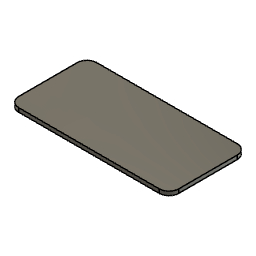
VFD_NTP_CLOCK_PLATE_T_V1.0 v3 (Autodesk Fusion 360 design; units mm, degrees)
Autodesk Fusion 360 part; units mm, degrees
sketch "スケッチ1" plane through (0, 0, 0) normal (0, 1, 0) x (1, 0, 0)
  line L0 (-41, 15) -> (-41, -15)
  line L1 (-36, 20) -> (36, 20)
  line L2 (41, 15) -> (41, -15)
  line L3 (-36, -20) -> (36, -20)
  arc A0 (-41, -15) -> (-36, -20) centre (-36, -15) ccw
  arc A1 (-36, 20) -> (-41, 15) centre (-36, 15) ccw
  arc A2 (41, 15) -> (36, 20) centre (36, 15) ccw
  arc A3 (36, -20) -> (41, -15) centre (36, -15) ccw
  dimension "d1" = 30
  dimension "d2" = 72
  constraint vertical L0
  constraint horizontal L1
  constraint perpendicular L1 L2
  constraint perpendicular L2 L3
  constraint tangent L0 A0
  constraint tangent L0 A1
  constraint tangent L1 A2
  constraint tangent L2 A3
  measures "d1" distance of L0.start L0.end
  measures "d2" distance of L1.start L1.end
extrude "押し出し1" add sketch "スケッチ1" along normal blind 2
